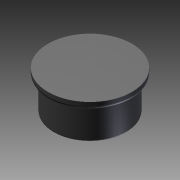
# Autodesk Inventor part: SB40-trmnl_hold
Saved by Autodesk Inventor 2014 (Build 180170000, 170)
## iProperties
Category: PARTsolutions
Company: NKKSWITCHES
Created: 2013-12-28
Part Number: SB40-trmnl_hold
Catalog Web Link: www.cadenas.de
Description: SB4011 Series - 3 Amp Momentary Pushbuttons -trmnl_hold-
Vendor: NKKSWITCHES
Document SubType Name: Modeling
Designer: PARTuser1
Manufacturer: NKKSWITCHES
Density: 1 g/cm^3
Material: Generic
Appearance: RGB(51.00000075995865,51.00000075995865,51.00000075995865)
PSOL_IDENT_0: {$CADENAS_DATA\23d-libs\nkkswitches\pushbuttons\sb4011\parts\sb4011_trmnls_hold.prj},221 {VTYP=3D},{
PSOL_IDENT_1: NB=SB40-trmnl_hold},{LINA=SB40-trmnl_hold},{NN=SB4011 Series - 3 Amp Momentary Pushbuttons -trmnl_ho
PSOL_IDENT_2: ld},{DATE=17.02.2009 10:23:06},{GEOMDATE=16.02.2009 10:08:00},{VERSION=},{LINEID=10},{LINESUBID=-1},
PSOL_IDENT_3: {WBVAR=}  {NB=SB40-trmnl_hold},{LINA=SB40-trmnl_hold},{KT=DUMMY},{PN=SB40},{SRS=SB40}
CNS_NN: SB4011 Series - 3 Amp Momentary Pushbuttons -trmnl_hold
CNS_NB: SB40-trmnl_hold
CNS_NBSYN: $PN.-trmnl_hold
CNS_LINA: SB40-trmnl_hold
CNS_PN: SB40
CNS_SRS: SB40
SUPPLIER: NKKSWITCHES
ARTICLENO: SB40-trmnl_hold
BOMINFO: SB40-trmnl_hold
CREATOR: CADENAS GmbH
Title: SB40-trmnl_hold
Author: Cadenas PARTsolutions
Autodesk Inventor part; units mm, degrees
sketch "Sketch_2" plane through (0, 0, 0) normal (1, 0, 0) x (0, 1, 0)
  line L0 (-3.9878, 0) -> (0, 0)
  line L1 (0, 0) -> (0, -5.0038)
  line L2 (0, -5.0038) -> (-3.7338, -5.0038)
  arc A0 (-3.9878, -4.7498) -> (-3.7338, -5.0038) centre (-3.7338, -4.7498) ccw
  line L3 (-3.9878, -4.7498) -> (-3.9878, 0)
  line L4 (-3.9878, 0) -> (0, 0)
  constraints: 10 end point, 2 point on circle, 1 centre point
revolve "Revolution1" add sketch "Sketch_2" angle 360 about axis through (0, -3.9878, 0) along (0, -1, 0)
sketch "Sketch_4" plane through (0, 0, 0) normal (1, 0, 0) x (0, 1, 0)
  line L0 (-0.254, 0) -> (1.27, 0)
  line L1 (1.27, 0) -> (1.27, -5.7404)
  line L2 (1.27, -5.7404) -> (0.762, -5.7404)
  arc A0 (0.254, -5.2324) -> (0.762, -5.7404) centre (0.762, -5.2324) ccw
  line L3 (0.254, -5.2324) -> (0.254, -4.9784)
  line L4 (0.254, -4.9784) -> (-0.254, -4.9784)
  line L5 (-0.254, -4.9784) -> (-0.254, 0)
  line L6 (-0.254, 0) -> (1.27, 0)
  constraints: 14 end point, 2 point on circle, 1 centre point
revolve "Revolution2" add sketch "Sketch_4" angle 360 about axis through (0, -0.254, 0) along (0, -1, 0)
ref_plane "to_body_XY" through (0, 0, 0) normal (0, -1, 0) x (1, 0, 0)
ref_plane "to_body_YZ" through (0, 0, 0) normal (1, 0, 0) x (0, 0, 1)
ref_plane "to_body_ZX" through (0, 0, 0) normal (0, 0, 1) x (0, -1, 0)
ref_plane "to_trmnls_XY" through (0, -3.7338, 0) normal (0, 1, 0) x (1, 0, 0)
ref_plane "to_trmnls_YZ" through (0, -3.7338, 0) normal (1, 0, 0) x (0, 0, -1)
ref_plane "to_trmnls_ZX" through (0, -3.7338, 0) normal (0, 0, -1) x (0, 1, 0)
body "Solid1"
